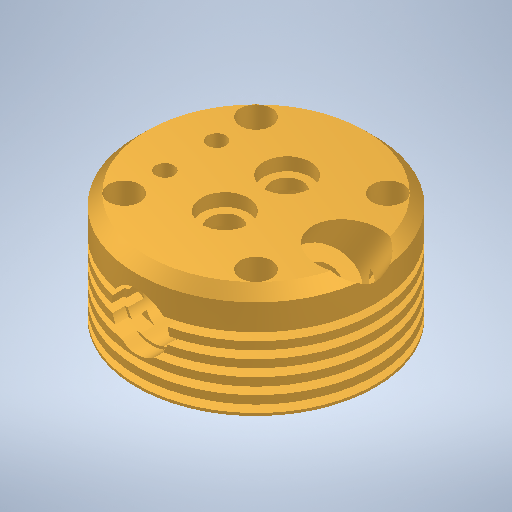
# Autodesk Inventor part: deckeGehaeuse
Saved by Autodesk Inventor 2025 (Build 290162010, 162A)
## iProperties
Created: 2024-07-15
Part Number: deckeGehaeuse
Material: Brass, Soft Yellow
Document SubType Name: Modeling
Designer: Fabri
Density: 8.47 g/cm^3
Appearance: Brass - Satin
Author: Fabri
Autodesk Inventor part; units mm, degrees
note: some values were not read from the file. Chosen so that the rebuilt part matches the saved one: direction of "Hole6".
sketch "Sketch1" plane through (0, 0, 0) normal (0, 1, 0) x (-1, 0, 0)
  line L0 (0, 0) -> (0, 21)
  line L1 (0, 21) -> (-23, 21)
  line L2 (-23, 21) -> (-23, 0)
  line L3 (-23, 0) -> (0, 0)
  dimension "d0" = 46
  dimension "d1" = 21
  constraints: 8 end point, 3 perpendicular, 1 vertical
  measures "d0" diameter of L2 L0
  measures "d1" distance between parallel lines of L3 L1
revolve "Revolution1" add sketch "Sketch1" angle 360 about axis through (0, 0, 0) along (0, 0, 1)
ref_plane "Work Plane1" through (0, 0, 0) normal (1, 0, 0) x (0, 1, 0)
sketch "Sketch3" plane through (0, 0, 0) normal (1, 0, 0) x (0, 1, 0)
  line L0 (23, 0) -> (-23, 0) projected
  line L1 (23, 21) -> (-23, 21) projected
  line L2 (0, 0) -> (0, 21)
  line L3 (23, 0) -> (23, 21) projected
  line L4 (23, 14) -> (17.5499, 14)
  line L5 (17.5499, 14) -> (17.5499, 12.5)
  line L6 (17.5499, 12.5) -> (23, 12.5)
  line L7 (23, 11) -> (17.5499, 11)
  line L8 (17.5499, 11) -> (17.5499, 9.5)
  line L9 (17.5499, 9.5) -> (23, 9.5)
  line L10 (23, 8) -> (17.5499, 8)
  line L11 (17.5499, 8) -> (17.5499, 6.5)
  line L12 (17.5499, 6.5) -> (23, 6.5)
  line L13 (23, 5) -> (21, 5)
  line L14 (21, 5) -> (21, 3.5)
  line L15 (21, 3.5) -> (23, 3.5)
  line L16 (23, 2) -> (21, 2)
  line L17 (21, 2) -> (21, 0.5)
  line L18 (21, 0.5) -> (23, 0.5)
  point P0 (0, 10.5)
  point P1 (22, 5)
  dimension "d16" = 1.5
  dimension "d17" = 1.5
  dimension "d18" = 1.5
  dimension "d19" = 1.5
  dimension "d20" = 1.5
  dimension "d21" = 36
  dimension "d22" = 6.5
  dimension "d23" = 1.5
  dimension "d24" = 1.5
  dimension "d25" = 1.5
  dimension "d26" = 1.5
  dimension "d27" = 42
  constraints: 32 end point, 8 horizontal, 6 point on line, 3 midpoint, 3 perpendicular, 3 vertical alignment, 1 parallel, 11 other
  measures "d16" distance between parallel lines of L6 L4
  measures "d17" distance between parallel lines of L7 L6
  measures "d18" distance between parallel lines of L7 L9
  measures "d19" distance between parallel lines of L10 L9
  measures "d20" distance between parallel lines of L12 L10
  measures "d21" diameter of L11.end point (0, 10.5)
  measures "d22" distance between parallel lines of L0 L12
  measures "d23" distance from line of point (22, 5) L12
  measures "d24" distance between parallel lines of L15 L13
  measures "d25" distance between parallel lines of L16 L15
  measures "d26" distance between parallel lines of L18 L16
  measures "d27" diameter of L14 L2
revolve "Revolution2" cut sketch "Sketch3" angle 360 about axis through (0, 0, 0) along (0, 0, 1) contours L18 L17 L16 L3 | L15 L14 L13 L3 | L3 L6 L5 L4 | L12 L11 L10 L3 | L3 L9 L8 L7
ref_plane "Work Plane10" through (0, 0, 21) normal (0, 0, 1) x (1, 0, 0)
sketch "Sketch12" plane through (0, 0, 21) normal (0, 0, 1) x (1, 0, 0)
  point P0 (0, 6)
  point P1 (0, -6)
  point P2 (0, 0)
  dimension "d64" = 12
  measures "d64" distance of point (0, -6) point (0, 6)
hole "Hole2" at (0, 6, 21) at (0, -6, 21) direction (0, 0, -1) diameter 6 depth 4.5 counterbore diameter 9 counterbore depth 2.5
sketch "Sketch13" plane through (0, 0, 21) normal (0, 0, 1) x (1, 0, 0)
  circle A0 centre (0, 0) radius 18 construction
  line L0 (0, 0) -> (-12.7279, -12.7279) construction
  line L1 (0, 0) -> (-18, 0) construction
  dimension "d72" = 36
  dimension "d73" = 45
  constraints: 4 end point, 2 point on circle, 1 centre point, 1 coincident, 1 horizontal
  measures "d72" diameter of A0
  measures "d73" angle of L1 L0
hole "Hole3" at (-12.7279, -12.7279, 21) direction (0, 0, -1) diameter 6 depth 5
pattern_circular "Circular Pattern1" count 4 over 360 about axis through (0, 0, 10.5) along (0, 0, 1) of "Hole3"
ref_plane "Work Plane11" through (0, 0, 16.5) normal (0, 0, 1) x (1, 0, 0)
sketch "Sketch14" plane through (0, 0, 16.5) normal (0, 0, 1) x (1, 0, 0)
  point P0 (0, 6)
  point P1 (0, -6)
  point P2 (0, 0)
  dimension "d93" = 12
  measures "d93" distance of point (0, -6) point (0, 6)
hole "Hole4" at (0, 6, 16.5) at (0, -6, 16.5) direction (0, 0, -1) diameter 11 depth 12
sketch "Sketch16" plane through (0, 0, 0) normal (1, 0, 0) x (0, 1, 0)
  line L0 (0, 0) -> (0, 4.5)
  line L1 (0, 4.5) -> (11.5, 4.5)
  line L2 (11.5, 4.5) -> (11.5, 2)
  line L3 (-21, 2) -> (21, 2) projected
  line L4 (11.5, 2) -> (14.5, 2)
  line L5 (14.5, 2) -> (14.5, 0)
  line L6 (14.5, 0) -> (0, 0)
  line L7 (11.5, 4.5) -> (11.5, 16.5) projected
  line L8 (11.5, 2) -> (14.5, 2)
  dimension "d94" = 2
  dimension "d95" = 2.5
  dimension "d96" = 29
  constraints: 14 end point, 5 perpendicular, 1 coincident, 1 collinear, 1 vertical
  measures "d94" distance between parallel lines of L6 L4
  measures "d95" distance between parallel lines of L4 L1
  measures "d96" diameter of L5 L0
revolve "Revolution4" cut sketch "Sketch16" angle 360 about axis through (0, 0, 0) along (0, 0, -1)
ref_plane "Work Plane6" through (0, 23, 0) normal (0, 1, 0) x (-1, 0, 0)
sketch "Sketch18" plane through (0, 23, 0) normal (0, 1, 0) x (-1, 0, 0)
  line L0 (23, 21) -> (-23, 21) projected
  line L1 (23, 0) -> (-23, 0) construction
  point P0 (0, 0)
  point P1 (0, 11)
  dimension "d161" = 11
  constraints: 1 vertical alignment
  measures "d161" distance from line of L1 point (0, 11)
hole "Hole5" at (0, 23, 11) direction (0, -1, 0) diameter 10 depth 13 counterbore diameter 11 counterbore depth 3
mirror "Mirror2" about plane through (0, 0, 0) normal (0, 1, 0) of "Hole5"
ref_plane "Work Plane7" through (0, 0, 0) normal (0, 1, 0) x (-1, 0, 0)
sketch "Sketch20" plane through (0, 0, 0) normal (0, 1, 0) x (-1, 0, 0)
  line L0 (0, 0) -> (0, 25.5973) construction
  line L1 (-7.6897, 4.5) -> (-18, 21)
  line L2 (14.5, 0) -> (-14.5, 0) projected
  line L3 (-9.7279, 21) -> (-9.7279, 21) projected
  line L4 (-11.5, 4.5) -> (0, 4.5) projected
  line L5 (-11.2272, 4.5) -> (-15.377, 11.1411)
  line L6 (-15.377, 11.1411) -> (-17.9212, 9.5514)
  line L7 (-17.9212, 9.5514) -> (-25.0751, 21)
  line L8 (23, 21) -> (-23, 21) projected
  line L9 (-18, 21) -> (-23, 21)
  line L10 (-25.0751, 21) -> (-18, 21)
  dimension "d127" = 18
  dimension "d137" = 122
  dimension "d138" = 12
  dimension "d139" = 6
  dimension "d148" = 13.5
  constraints: 15 end point, 2 parallel, 2 point on line, 1 collinear, 1 horizontal, 1 horizontal alignment, 1 perpendicular, 1 vertical
  measures "d127" distance from line of L0 L1.end
  measures "d137" angle of L2 L1
  measures "d138" diameter of L7.end L1
  measures "d139" diameter of L5 L1
  measures "d148" distance of L6.end L7.end
revolve "Revolution6" cut sketch "Sketch20" angle 360 about axis through (7.6897, 0, 4.5) along (-0.5299193, 0, -0.8480481)
chamfer "Chamfer2" distance 2 angle 45 1 edges at (-23, 0, 21)
sketch "Sketch22" plane through (0, 0, 21) normal (0, 0, 1) x (1, 0, 0)
  point P0 (0, 0)
  point P1 (-12.6, 5)
  point P2 (-12.6, -5)
  dimension "d151" = 12.6
  dimension "d152" = 5
  dimension "d153" = 5
  constraints: 1 vertical alignment
  measures "d151" horizontal distance of point (-12.6, 5) point (0, 0)
  measures "d152" vertical distance of point (0, 0) point (-12.6, 5)
  measures "d153" vertical distance of point (0, 0) point (-12.6, -5)
hole "Hole6" at (-12.6, 5, 21) at (-12.6, -5, 21) direction (0, 0, -1) diameter 3.5 depth 7
equation "\"d17\" = d16"
equation "\"d18\" = d16"
equation "\"d19\" = d16"
equation "\"d20\" = d16"
equation "\"d24\" = d23"
equation "\"d25\" = d23"
equation "\"d26\" = d23"
equation "\"d153\" = d152"
body "Solid1"
